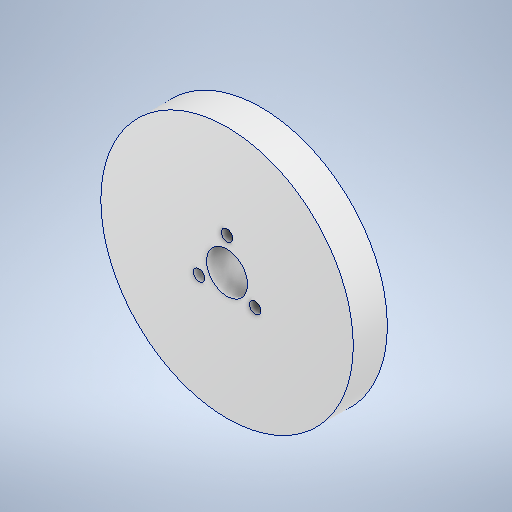
# Autodesk Inventor part: rotor_hub
Saved by Autodesk Inventor 2025.2 (Build 292293000, 293)
## iProperties
Created: 2025-03-04
Part Number: rotor_hub
Material: Aluminum 6061
Document SubType Name: Modeling
Designer: aaron
Density: 2.7 g/cm^3
Appearance: Aluminum - Flat
Author: aaron
Autodesk Inventor part; units mm, degrees
ref_plane "YZ Plane" through (0, 0, 0) normal (1, 0, 0) x (0, 1, 0)
ref_plane "XZ Plane" through (0, 0, 0) normal (0, 1, 0) x (-1, 0, 0)
ref_plane "XY Plane" through (0, 0, 0) normal (0, 0, 1) x (1, 0, 0)
sketch "Sketch1" plane through (0, 0, 0) normal (0, 0, 1) x (1, 0, 0)
  circle A0 centre (0, 0) radius 37
  dimension "d0" = 74
  constraints: 1 centre point, 1 coincident
  measures "d0" diameter of A0
extrude "Extrusion1" add sketch "Sketch1" along normal blind 10
sketch "Sketch4" plane through (0, 0, 0) normal (0, 0, -1) x (-1, 0, 0)
  circle A0 centre (0, 0) radius 29
  circle A1 centre (0, 0) radius 17
  circle A2 centre (0, 0) radius 37 projected
  dimension "d5" = 8
  dimension "d6" = 34
  constraints: 2 centre point, 2 coincident
  measures "d5" radial gap between concentric circles of A0 A2
  measures "d6" diameter of A1
extrude "Extrusion3" cut sketch "Sketch4" against normal blind 6 contours A0
sketch "Sketch6" plane through (0, 0, 0) normal (0, 0, -1) x (-1, 0, 0)
  circle A0 centre (0, 0) radius 15
  dimension "d9" = 30
  constraints: 1 centre point, 1 coincident
  measures "d9" diameter of A0
extrude "Extrusion4" add sketch "Sketch6" along normal blind 7
sketch "Sketch8" plane through (0, 0, -7) normal (0, 0, -1) x (-1, 0, 0)
  circle A0 centre (0, 0) radius 9.5
  circle A1 centre (0, 9.5) radius 1.65
  circle A2 centre (-8.2272, -4.75) radius 1.65
  circle A3 centre (8.2272, -4.75) radius 1.65
  circle A4 centre (0, 0) radius 6
  dimension "d16" = 19
  dimension "d17" = 3.3
  dimension "d20" = 360
  dimension "d24" = 12
  constraints: 4 centre point, 2 coincident, 1 vertical alignment, 9 other
  measures "d17" diameter of A1
  measures "d24" diameter of A4
extrude "Extrusion6" cut sketch "Sketch8" against normal through all contours A1 A0 | A0 A1 | A3 A0 | A0 A3 | A2 A0 | A0 A2 | A4
body "Solid1"
